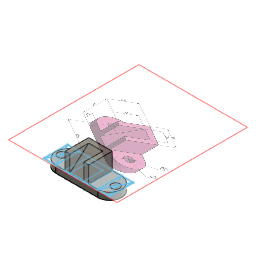
A2 v1 (Autodesk Fusion 360 design; units mm, degrees)
Autodesk Fusion 360 part; units mm, degrees
sketch "Sketch1" plane through (0, 0, 0) normal (0, 1, 0) x (1, 0, 0)
  line L0 (-23.7399, -107.7068) -> (90.2601, -107.7068)
  line L1 (90.2601, -107.7068) -> (90.2601, -171.7068)
  line L2 (90.2601, -171.7068) -> (-23.7399, -171.7068)
  line L3 (-23.7399, -171.7068) -> (-23.7399, -107.7068)
  line L4 (-23.7399, -171.7068) -> (-55.7399, -171.7068)
  line L5 (-55.7399, -171.7068) -> (-55.7399, -107.7068)
  line L6 (-55.7399, -107.7068) -> (-23.7399, -107.7068)
  line L7 (90.2601, -171.7068) -> (122.2601, -171.7068)
  line L8 (1.2601, -107.7068) -> (1.2601, -171.7068)
  line L9 (65.2601, -107.7068) -> (65.2601, -171.7068)
  line L10 (122.2601, -171.7068) -> (122.2601, -107.7068)
  line L11 (122.2601, -107.7068) -> (90.2601, -107.7068)
  line L12 (-55.7399, -107.7068) -> (-23.7399, -171.7068)
  line L13 (-23.7399, -107.7068) -> (-55.7399, -171.7068)
  line L14 (90.2601, -107.7068) -> (122.2601, -171.7068)
  line L15 (90.2601, -171.7068) -> (122.2601, -107.7068)
  line L16 (14.2601, -171.7068) -> (52.2601, -171.7068)
  line L17 (52.2601, -171.7068) -> (52.2601, -120.7068)
  line L18 (52.2601, -120.7068) -> (14.2601, -120.7068)
  line L19 (14.2601, -120.7068) -> (14.2601, -171.7068)
  dimension "d1" = 114
  dimension "d2" = 64
  dimension "d3" = 32
  dimension "d4" = 32
  dimension "d5" = 64
  dimension "d6" = 25
  dimension "d7" = 25
  dimension "d8" = 13
  dimension "d9" = 13
  dimension "d10" = 13
  dimension "d11" = 51
  dimension "d12" = 38
  constraint horizontal L0
  constraint vertical L1
  constraint horizontal L2
  constraint vertical L3
  constraint perpendicular L3 L4
  constraint perpendicular L4 L5
  constraint perpendicular L3 L6
  constraint perpendicular L1 L7
  constraint coincident L0 L8.start
  constraint coincident L2 L8.end
  constraint perpendicular L2 L8
  constraint coincident L0 L9.start
  constraint coincident L2 L9.end
  constraint perpendicular L2 L9
  constraint perpendicular L7 L10
  constraint perpendicular L10 L11
  constraint perpendicular L16 L17
  constraint parallel L16 L18
  constraint parallel L17 L19
  constraint coincident L2 L16.end
  constraint perpendicular L8 L16
  measures "d1" distance of L0.start L0.end
  measures "d2" distance of L0.start L2.end
  measures "d3" distance of L2.end L4.end
  measures "d4" distance of L1.end L7.end
  measures "d5" distance of L8 L9
  measures "d6" distance of L3 L8
  measures "d7" distance of L1 L9
  measures "d8" distance of L8 L19
  measures "d9" distance of L9 L17
  measures "d10" distance of L0 L18
  measures "d11" distance of L16 L18
  measures "d12" distance of L17 L19
extrude "Extrude1" add sketch "Sketch1" against normal blind 19
hole "Hole1" at (-39.7798, 0, 139.6675) direction (0, -1, 0) diameter 22 depth 19 tip angle 118
hole "Hole2" at (106.2375, 0, 139.7024) direction (0, -1, 0) diameter 22 depth 19 tip angle 118
extrude "Extrude2" add sketch "Sketch1" along normal blind 45 contours L0 L2 L8 L9 L17 L18 L19
draft "Draft1" angle 41.45 neutral plane through (14.2601, 0, 171.7068) pull (0, 0, 1) 1 faces at (26.9268, 0, 154.7068)
fillet "Fillet1" radius 32 1 edges at (122.2601, -9.5, 171.7068)
fillet "Fillet2" radius 32 1 edges at (122.2601, -9.5, 107.7068)
fillet "Fillet3" radius 32 1 edges at (-55.7399, -9.5, 171.7068)
fillet "Fillet4" radius 32 1 edges at (-55.7399, -9.5, 107.7068)
equation "d6 = ( ( 114 - 64 ) / 2 ) * 1 mm"
equation "d21 = 64 mm - 19 mm"
named bodies: "A2"
